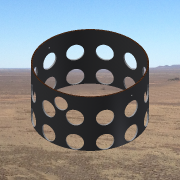
# Autodesk Inventor part: 2h2sono
Saved by Autodesk Inventor 2013 SP2 (Build 170200200, 200)
## iProperties
Company: HERA Project
Created: 2013-05-14
Part Number: 2h2sono
Material: Generic
Document SubType Name: Modeling
Designer: David DeBoer
Density: 1 g/cm^3
Description: Hub inner sonotube
Mass: 1625.04 g
Surface Area: 5665.19 cm^2
Volume: 1625.04 cm^3
Author: David DeBoer
Title: Hub innersono
Autodesk Inventor part; units mm, degrees
ref_plane "YZ Plane" through (0, 0, 0) normal (1, 0, 0) x (0, 1, 0)
ref_plane "XZ Plane" through (0, 0, 0) normal (0, 1, 0) x (-1, 0, 0)
ref_plane "XY Plane" through (0, 0, 0) normal (0, 0, 1) x (1, 0, 0)
sketch "Sketch1" plane through (0, 0, 0) normal (0, 1, 0) x (-1, 0, 0)
  circle A0 centre (0, 0) radius 228.6
  circle A1 centre (0, 0) radius 222.25
  dimension "d0" = 457.2
  dimension "d2" = 6.35
  constraints: 2 centre point, 1 coincident
  measures "d0" diameter of A0
  measures "d2" radial gap between concentric circles of A1 A0
extrude "tube" add sketch "Sketch1" along normal blind 254
sketch "Sketch2" plane through (0, 254, 0) normal (0, 1, 0) x (1, 0, 0)
  circle A0 centre (0, 0) radius 222.25 projected
  circle A1 centre (0, 0) radius 228.6 projected
  point P0 (-228.6, 0)
  constraints: 1 horizontal alignment, 1 other
ref_plane "Work Plane1" through (-228.6, 254, 0) normal (-1, 0, 0) x (0, -1, 0)
sketch "Sketch3" plane through (-228.6, 254, 0) normal (-1, 0, 0) x (0, -1, 0)
  circle A0 centre (101.6, 0) radius 25.4
  line L0 (254, -228.6) -> (254, 228.6) projected
  point P0 (254, 0)
  dimension "d5" = 50.8
  dimension "d36" = 152.4
  constraints: 1 centre point
  measures "d5" diameter of A0
  measures "d36" distance from line of A0.centre L0
hole "spar" at (-228.6, 152.4, 0) direction (1, 0, 0) diameter 73.025 end through all
pattern_circular "spar pattern" count 12 over 360 about axis through (0, 0, 0) along (0, 1, 0) of "spar"
sketch "Sketch7" plane through (0, 254, 0) normal (0, 1, 0) x (1, 0, 0)
  circle A0 centre (0, 0) radius 222.25 projected
  circle A1 centre (0, 0) radius 228.6 projected
  line L0 (0, 0) -> (297.2113, -59.119) construction
  line L1 (0, 0) -> (303.0341, 0) construction
  point P0 (224.2075, -44.5976)
  dimension "d45" = 11.25
  constraints: 4 end point, 1 equal length, 1 horizontal, 1 point on line, 2 other
  measures "d45" angle of L0 L1
ref_plane "Work Plane2" through (224.2075, 254, 44.5976) normal (0.9807853, 0, 0.1950903) x (0, 1, 0)
sketch "Sketch10" plane through (-228.6, 254, 0) normal (-1, 0, 0) x (0, -1, 0)
  circle A0 centre (215.9, 0) radius 30.1625
  point P0 (254, 0)
  dimension "d62" = 60.325
  dimension "d63" = 38.1
  constraints: 1 centre point
  measures "d62" diameter of A0
  measures "d63" distance of point (254, 0) A0.centre
hole "support" at (-228.6, 38.1, 0) direction (1, 0, 0) diameter 73.025 end through all
pattern_circular "support pattern" count 12 over 360 about axis through (0, 0, 0) along (0, 1, 0) of "support"
sketch "Sketch11" plane through (0, 254, 0) normal (0, 1, 0) x (1, 0, 0)
  circle A0 centre (0, 0) radius 222.25 projected
  circle A1 centre (0, 0) radius 228.6 projected
  point P0 (60.0075, -220.5835)
  constraints: 2 other
ref_plane "Work Plane3" through (60.0075, 254, 220.5835) normal (0.2625, 0, 0.964932) x (0, 1, 0)
sketch "Sketch12" plane through (60.0075, 254, 220.5835) normal (0.2625, 0, 0.964932) x (0, 1, 0)
  circle A0 centre (-50.8, 0) radius 30.48
  point P0 (-254, 0)
  dimension "d74" = 60.96
  dimension "d76" = 203.2
  constraints: 1 centre point
  measures "d74" diameter of A0
  measures "d76" distance of point (-254, 0) A0.centre
extrude "conduit" cut sketch "Sketch12" against normal blind 25.4
sketch "Sketch15" plane through (0, 254, 0) normal (0, 1, 0) x (1, 0, 0)
  circle A0 centre (0, 0) radius 222.25 projected
  circle A1 centre (0, 0) radius 228.6 projected
  point P0 (-214.141, -80.01)
  constraints: 2 other
ref_plane "Work Plane5" through (-214.141, 254, 80.01) normal (-0.9367497, 0, 0.35) x (0, -1, 0)
sketch "Sketch17" plane through (0, 254, 0) normal (0, 1, 0) x (1, 0, 0)
  circle A0 centre (0, 0) radius 222.25 projected
  circle A1 centre (0, 0) radius 228.6 projected
  point P0 (-228.6, 0)
  constraints: 1 horizontal alignment, 1 other
ref_plane "Work Plane6" through (-228.6, 254, 0) normal (-1, 0, 0) x (0, -1, 0)
sketch "Sketch18" plane through (-228.6, 254, 0) normal (-1, 0, 0) x (0, -1, 0)
  circle A0 centre (38.1, 0) radius 6.35
  line L0 (0, 228.6) -> (0, -228.6) projected
  point P0 (254, 0)
  dimension "d88" = 12.7
  dimension "d89" = 38.1
  constraints: 1 centre point
  measures "d88" diameter of A0
  measures "d89" distance from line of A0.centre L0
hole "Hole8" at (-228.6, 215.9, 0) direction (1, 0, 0) diameter 6.35 end through all
body "Solid1"
